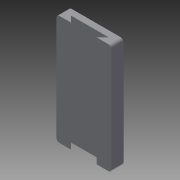
# Autodesk Inventor part: nano_enclosure_modular_sidelock
Saved by Autodesk Inventor 2015 (Build 190159000, 159)
## iProperties
Created: 2015-02-26
Part Number: nano_enclosure_modular_sidelock
Material: Generic
Document SubType Name: Modeling
Designer: Jeff
Density: 1 g/cm^3
Appearance: Default
Author: Jeff
Autodesk Inventor part; units mm, degrees
ref_plane "YZ Plane" through (0, 0, 0) normal (1, 0, 0) x (0, 1, 0)
ref_plane "XZ Plane" through (0, 0, 0) normal (0, 1, 0) x (-1, 0, 0)
ref_plane "XY Plane" through (0, 0, 0) normal (0, 0, 1) x (1, 0, 0)
sketch "Sketch1" plane through (0, 0, 0) normal (0, 0, 1) x (1, 0, 0)
  line L0 (0, 0) -> (22.86, 0)
  line L1 (22.86, 0) -> (22.86, 45.72)
  line L2 (22.86, 45.72) -> (0, 45.72)
  line L3 (0, 45.72) -> (0, 0)
  dimension "d0" = 22.86
  dimension "d1" = 45.72
  constraints: 8 end point, 2 parallel, 1 horizontal, 1 perpendicular
  measures "d0" distance of L2.end L1.end
  measures "d1" distance of L0.end L1.end
extrude "Extrusion1" add sketch "Sketch1" along normal blind 5.08
sketch "Sketch2" plane through (0, 0, 0) normal (0, -1, 0) x (1, 0, 0)
  line L0 (0, 5.08) -> (22.86, 5.08) projected
  line L1 (6.096, 5.08) -> (3.556, 2.54)
  line L2 (3.556, 2.54) -> (19.304, 2.54)
  line L3 (19.304, 2.54) -> (16.764, 5.08)
  line L4 (6.096, 5.08) -> (16.764, 5.08)
  line L5 (0, 0) -> (0, 5.08) projected
  line L6 (0, 0) -> (22.86, 0) projected
  dimension "d4" = 45
  dimension "d5" = 45
  dimension "d6" = 10.668
  dimension "d7" = 3.556
  dimension "d8" = 2.54
  dimension "d12" = 2.54
  constraints: 8 end point, 2 point on line, 1 collinear, 1 parallel
  measures "d4" angle of L2 L1
  measures "d5" angle of L2 L3
  measures "d6" distance of L3.end L1.start
  measures "d7" distance from line of L5 L1.end
  measures "d8" distance between parallel lines of L6 L2
  measures "d12" horizontal distance of L2.end L3.end
extrude "Extrusion2" cut sketch "Sketch2" against normal blind 50.8
fillet "Fillet1" radius 1.27 4 edges at (0, 0, 2.54) (22.86, 0, 2.54) (22.86, 45.72, 2.54) (0, 45.72, 2.54)
body "Solid1"
